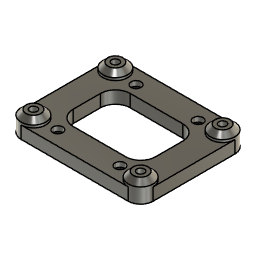
Din Mount Adapter (Autodesk Fusion 360 design; units mm, degrees)
Autodesk Fusion 360 part; units mm, degrees
note: some values were not read from the file. Set by a fixed rule: which sketch regions a step uses.
sketch "Sketch1" plane through (0, 0, 0) normal (0, 0, 1) x (1, 0, 0)
  line L0 (0, 0) -> (43.2, 0) construction
  line L1 (43.2, 0) -> (43.2, 33) construction
  line L2 (43.2, 33) -> (0, 33) construction
  line L3 (0, 33) -> (0, 0) construction
  circle A0 centre (0, 33) radius 2.35
  circle A1 centre (0, 0) radius 2.35
  circle A2 centre (43.2, 0) radius 2.35
  circle A3 centre (43.2, 33) radius 2.35
  line L4 (0, -5) -> (43.2, -5)
  line L5 (48.2, 0) -> (48.2, 33)
  line L6 (43.2, 38) -> (0, 38)
  line L7 (-5, 33) -> (-5, 0)
  arc A4 (0, 38) -> (-5, 33) centre (0, 33) ccw
  arc A5 (48.2, 33) -> (43.2, 38) centre (43.2, 33) ccw
  arc A6 (43.2, -5) -> (48.2, 0) centre (43.2, 0) ccw
  arc A7 (-5, 0) -> (0, -5) centre (0, 0) ccw
  circle A8 centre (0, 33) radius 5
  circle A9 centre (0, 0) radius 5
  circle A10 centre (43.2, 0) radius 5
  circle A11 centre (43.2, 33) radius 5
  line L8 (9.1, 32.25) -> (34.1, 32.25) construction
  line L9 (34.1, 32.25) -> (34.1, 0.75) construction
  line L10 (34.1, 0.75) -> (9.1, 0.75) construction
  line L11 (9.1, 0.75) -> (9.1, 32.25) construction
  line L12 (9.1, 0.75) -> (34.1, 32.25) construction
  line L13 (9.1, 32.25) -> (34.1, 0.75) construction
  line L14 (0, 0) -> (43.2, 33) construction
  line L15 (0, 33) -> (43.2, 0) construction
  circle A12 centre (9.1, 32.25) radius 1.2
  circle A13 centre (9.1, 0.75) radius 1.2
  circle A14 centre (34.1, 0.75) radius 1.2
  circle A15 centre (34.1, 32.25) radius 1.2
  circle A16 centre (9.1, 32.25) radius 2
  circle A17 centre (34.1, 32.25) radius 2
  circle A18 centre (9.1, 0.75) radius 2
  circle A19 centre (34.1, 0.75) radius 2
  line L16 (11, 5) -> (32.2, 5)
  line L17 (38.2, 11) -> (38.2, 22)
  line L18 (32.2, 28) -> (11, 28)
  line L19 (5, 22) -> (5, 11)
  arc A20 (11, 28) -> (5, 22) centre (11, 22) ccw
  arc A21 (5, 11) -> (11, 5) centre (11, 11) ccw
  arc A22 (38.2, 22) -> (32.2, 28) centre (32.2, 22) ccw
  arc A23 (32.2, 5) -> (38.2, 11) centre (32.2, 11) ccw
  circle A24 centre (0, 33) radius 1.5
  circle A25 centre (43.2, 33) radius 1.5
  circle A26 centre (0, 0) radius 1.5
  circle A27 centre (43.2, 0) radius 1.5
  point P0 (21.6, 16.5)
  point P1 (21.6, 16.5)
  dimension "d1" = 43.2
  dimension "d2" = 33
  dimension "d3" = 4.7
  dimension "d4" = 4.7
  dimension "d5" = 4.7
  dimension "d6" = 4.7
  dimension "d8" = 5
  dimension "d9" = 10
  dimension "d10" = 10
  dimension "d11" = 10
  dimension "d12" = 10
  dimension "d13" = 25
  dimension "d14" = 31.5
  dimension "d15" = 2.4
  dimension "d16" = 2.4
  dimension "d17" = 2.4
  dimension "d18" = 2.4
  dimension "d19" = 4
  dimension "d20" = 4
  dimension "d21" = 4
  dimension "d22" = 4
  dimension "d30" = 6
  dimension "d31" = 3
  dimension "d32" = 3
  dimension "d33" = 3
  dimension "d34" = 3
  constraint horizontal L0
  constraint vertical L1
  constraint horizontal L2
  constraint vertical L3
  constraint coincident L0.start L3.end
  constraint coincident L2.end L3.start
  constraint coincident L0.end L1.start
  constraint coincident L1.end L2.start
  constraint tangent L6 A4
  constraint tangent L7 A4
  constraint tangent L5 A5
  constraint tangent L6 A5
  constraint equal A4 A5
  constraint tangent L4 A6
  constraint tangent L5 A6
  constraint equal A4 A6
  constraint tangent L4 A7
  constraint tangent L7 A7
  constraint equal A4 A7
  constraint concentric A4 A8
  constraint concentric A2 A10
  constraint concentric A5 A11
  constraint horizontal L8
  constraint vertical L9
  constraint horizontal L10
  constraint vertical L11
  constraint midpoint L14 P1
  constraint midpoint L12 P1
  constraint coincident P1 P0
  constraint coincident L8.start L11.end
  constraint coincident L10.end L11.start
  constraint coincident L9.end L10.start
  constraint coincident L8.end L9.start
  constraint concentric A12 A16
  constraint concentric A15 A17
  constraint concentric A13 A18
  constraint concentric A14 A19
  constraint tangent L18 A20
  constraint tangent L19 A20
  constraint tangent L16 A21
  constraint tangent L19 A21
  constraint equal A20 A21
  constraint tangent L17 A22
  constraint tangent L18 A22
  constraint equal A20 A22
  constraint tangent L16 A23
  constraint tangent L17 A23
  constraint equal A20 A23
  constraint concentric A8 A24
  constraint concentric A5 A25
  constraint concentric A10 A27
  measures "d1" distance of L0.start L0.end
  measures "d2" distance of L0.start L2.end
  measures "d3" diameter of A0
  measures "d4" diameter of A1
  measures "d5" diameter of A2
  measures "d6" diameter of A3
  measures "d8" radius of A4
  measures "d9" diameter of A8
  measures "d10" diameter of A9
  measures "d11" diameter of A10
  measures "d12" diameter of A11
  measures "d13" distance of L8.start L8.end
  measures "d14" distance of L8.start L10.end
  measures "d15" diameter of A12
  measures "d16" diameter of A13
  measures "d17" diameter of A14
  measures "d18" diameter of A15
  measures "d19" diameter of A16
  measures "d20" diameter of A17
  measures "d21" diameter of A18
  measures "d22" diameter of A19
  measures "d30" radius of A20
  measures "d31" diameter of A24
  measures "d32" diameter of A25
  measures "d33" diameter of A26
  measures "d34" diameter of A27
extrude "Extrude1" add sketch "Sketch1" against normal blind 3 contours L4 L5 L6 L7 A8 A9 A10 A11 | A7 A9 | A6 A10 | A4 A8 | A5 A11 | A16 | A17 | A18 | A19
extrude "Extrude2" add sketch "Sketch1" along normal blind 2 contours L4 L5 L6 L7 A8 A9 A10 A11 | A7 A9 | A6 A10 | A4 A8 | A5 A11
extrude "Extrude3" add sketch "Sketch1" along normal blind 5 contours A0 | A1 | A2 | A3 | A7 A9 | A6 A10 | A4 A8 | A5 A11
move_face "OffsetFaces1" offset -2 4 faces at (42.3395, 1.873, 0) (2.0579, -0.1167, 0) (-2.0579, 32.8833, 0) (41.1477, 32.8087, 0)
chamfer "Chamfer1" distance 0.5 angle 45 4 edges at (-2.191, -0.8498, -3) (41.009, -0.8498, -3) (41.009, 32.1502, -3) (-2.191, 32.1502, -3)
chamfer "Chamfer2" distance 2 angle 45 4 edges at (-4.6616, 31.1919, 5) (-4.6616, -1.8081, 5) (38.5384, -1.8081, 5) (38.5384, 31.1919, 5)
sketch "Sketch2" plane through (0, 0, 2) normal (0, 0, -1) x (1, 0, 0)
  circle A0 centre (0, 0) radius 1.5
  circle A1 centre (0, 0) radius 2.35
  line L0 (-1.5, 2.5) -> (1.5, 2.5)
  line L1 (1.5, 2.5) -> (1.5, -2.5)
  line L2 (1.5, -2.5) -> (-1.5, -2.5)
  line L3 (-1.5, -2.5) -> (-1.5, 2.5)
  line L4 (-1.5, -2.5) -> (1.5, 2.5) construction
  line L5 (-1.5, 2.5) -> (1.5, -2.5) construction
  line L6 (44.7, 2.5) -> (44.7, -2.5)
  line L7 (41.7, -2.5) -> (41.7, 2.5)
  line L8 (41.7, 2.5) -> (44.7, -2.5) construction
  line L9 (41.7, 2.5) -> (44.7, 2.5)
  line L10 (44.7, -2.5) -> (41.7, -2.5)
  line L11 (41.7, -2.5) -> (44.7, 2.5) construction
  circle A2 centre (0, -33) radius 1.5
  circle A3 centre (0, -33) radius 2.35
  circle A4 centre (43.2, -33) radius 1.5
  circle A5 centre (43.2, -33) radius 2.35
  circle A6 centre (43.2, 0) radius 1.5
  circle A7 centre (43.2, 0) radius 2.35
  line L12 (41.7, 2.5) -> (44.7, 2.5)
  line L13 (44.7, 2.5) -> (44.7, -2.5)
  line L14 (41.7, -2.5) -> (41.7, 2.5)
  line L15 (41.7, -2.5) -> (44.7, 2.5) construction
  line L16 (44.7, -2.5) -> (41.7, -2.5)
  line L17 (41.7, 2.5) -> (44.7, -2.5) construction
  line L18 (-1.5, -30.5) -> (1.5, -30.5)
  line L19 (1.5, -30.5) -> (1.5, -35.5)
  line L20 (-1.5, -35.5) -> (-1.5, -30.5)
  line L21 (-1.5, -35.5) -> (1.5, -30.5) construction
  line L22 (1.5, -35.5) -> (-1.5, -35.5)
  line L23 (-1.5, -30.5) -> (1.5, -35.5) construction
  line L24 (41.7, -30.5) -> (44.7, -35.5) construction
  line L25 (44.7, -30.5) -> (44.7, -35.5)
  line L26 (41.7, -30.5) -> (44.7, -30.5)
  line L27 (41.7, -30.5) -> (44.7, -35.5) construction
  line L28 (41.7, -35.5) -> (44.7, -30.5) construction
  line L29 (44.7, -35.5) -> (41.7, -35.5)
  line L30 (41.7, -35.5) -> (44.7, -30.5) construction
  line L31 (44.7, -35.5) -> (41.7, -35.5)
  line L32 (41.7, -30.5) -> (44.7, -30.5)
  line L33 (44.7, -30.5) -> (44.7, -35.5)
  line L34 (41.7, -35.5) -> (41.7, -30.5)
  line L35 (41.7, -35.5) -> (41.7, -30.5)
  point P0 (43.2, 0)
  point P1 (43.2, 0)
  point P2 (0, -33)
  point P3 (43.2, -33)
  point P4 (43.2, -33)
  dimension "d38" = 3
  dimension "d39" = 5
  dimension "d40" = 3
  dimension "d41" = 5
  dimension "d42" = 3
  dimension "d43" = 5
  dimension "d44" = 3
  dimension "d45" = 5
  dimension "d46" = 3
  dimension "d47" = 5
  dimension "d48" = 3
  dimension "d49" = 5
  constraint horizontal L0
  constraint vertical L1
  constraint horizontal L2
  constraint vertical L3
  constraint midpoint L5 A0.centre
  constraint coincident A0.centre A1.centre
  constraint horizontal L9
  constraint vertical L6
  constraint horizontal L10
  constraint vertical L7
  constraint midpoint P1 L8
  constraint horizontal L12
  constraint vertical L13
  constraint horizontal L16
  constraint vertical L14
  constraint midpoint P1 L17
  constraint horizontal L18
  constraint vertical L19
  constraint horizontal L22
  constraint vertical L20
  constraint midpoint P2 L23
  constraint horizontal L32
  constraint vertical L25
  constraint horizontal L29
  constraint vertical L35
  constraint midpoint P4 L27
  constraint horizontal L26
  constraint vertical L33
  constraint horizontal L31
  constraint vertical L34
  constraint midpoint P4 L24
  measures "d38" distance of L0.start L0.end
  measures "d39" distance of L0.start L2.end
  measures "d40" distance of L7.end L6.start
  measures "d41" distance of L7.end L7.start
  measures "d42" distance of L6.start L7.end
  measures "d43" distance of L7.start L7.end
  measures "d44" distance of L18.start L18.end
  measures "d45" distance of L18.start L20.start
  measures "d46" distance of L25.start L24.start
  measures "d47" distance of L28.start L24.start
  measures "d48" distance of L24.start L25.start
  measures "d49" distance of L24.start L28.start
extrude "Extrude4" cut sketch "Sketch2" against normal blind 0.2 contours A0 A1 L1 L3 | A0 A1 L1 L3 | L6 L7 A6 A7 L13 L14 | L6 L7 A6 A7 L13 L14 | A2 A3 L19 L20 | A2 A3 L19 L20 | A4 A5 L25 L33 L34 L35 | A4 A5 L25 L33 L34 L35
